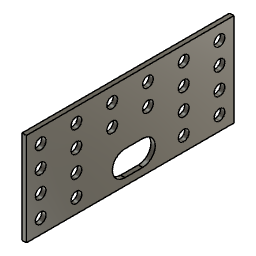
plate_4 v1 (Autodesk Fusion 360 design; units mm, degrees)
Autodesk Fusion 360 part; units mm, degrees
sketch "Sketch1" plane through (0, 0, 0) normal (1, 0, 0) x (0, 1, 0)
  line L0 (0, 0) -> (290.2, 0)
  line L1 (290.2, 0) -> (290.2, 130)
  line L2 (290.2, 130) -> (0, 130)
  line L3 (0, 130) -> (0, 0)
  dimension "d1" = 290.2
  dimension "d2" = 130
  constraint horizontal L0
  constraint vertical L1
  constraint horizontal L2
  constraint vertical L3
  constraint coincident L0.start L3.end
  measures "d1" distance of L0.start L0.end
  measures "d2" distance of L0.start L2.end
extrude "Extrude1" add sketch "Sketch1" against normal blind 6
sketch "Sketch2" plane through (0, 0, 0) normal (1, 0, 0) x (0, 1, 0)
  line L0 (0, 130) -> (0, 0)
  line L1 (0, 0) -> (290.2, 0)
  line L2 (290.2, 0) -> (290.2, 130)
  line L3 (290.2, 130) -> (0, 130)
  line L4 (162.7, 45) -> (137.7, 45)
  arc A0 (137.7, 45) -> (137.7, 10) centre (137.7, 27.5) ccw
  line L5 (137.7, 10) -> (162.7, 10)
  arc A1 (162.7, 10) -> (162.7, 45) centre (162.7, 27.5) ccw
  line L6 (180.2, 27.5) -> (120.2, 27.5) construction
  circle A2 centre (20, 110) radius 7.5
  circle A3 centre (70, 110) radius 7.5
  circle A4 centre (120, 110) radius 7.5
  circle A5 centre (170, 110) radius 7.5
  circle A6 centre (220, 110) radius 7.5
  circle A7 centre (270, 110) radius 7.5
  circle A8 centre (20, 80) radius 7.5
  circle A9 centre (70, 80) radius 7.5
  circle A10 centre (120, 80) radius 7.5
  circle A11 centre (170, 80) radius 7.5
  circle A12 centre (220, 80) radius 7.5
  circle A13 centre (270, 80) radius 7.5
  circle A14 centre (20, 50) radius 7.5
  circle A15 centre (70, 50) radius 7.5
  circle A16 centre (220, 50) radius 7.5
  circle A17 centre (270, 50) radius 7.5
  circle A18 centre (20, 20) radius 7.5
  circle A19 centre (70, 20) radius 7.5
  circle A20 centre (220, 20) radius 7.5
  circle A21 centre (270, 20) radius 7.5
  dimension "d5" = 35
  dimension "d6" = 110
  dimension "d7" = 10
  dimension "d8" = 15
  dimension "d9" = 20
  dimension "d10" = 20
  dimension "d13" = 250
  dimension "d14" = -90
  constraint tangent L4 A0
  constraint tangent A0 L5
  constraint parallel L4 L5
  constraint tangent L5 A1
  constraint tangent L4 A1
  constraint midpoint A1 L6.start
  constraint midpoint A0 L6.end
  constraint horizontal L6
  measures "d5" diameter of A0
  measures "d6" distance of L2 L6.start
  measures "d7" distance of L1 L5
  measures "d8" diameter of A2
  measures "d9" distance of L3 A2.centre
  measures "d10" distance of L0 A2.centre
extrude "Extrude2" cut sketch "Sketch2" against normal up to surface (6 mm away) contours L4 A0 L5 A1 | A2 | A3 | A4 | A5 | A6 | A7 | A8 | A9 | A10 | A11 | A12 | A13 | A14 | A15 | A16 | A17 | A18 | A19 | A20 | A21
